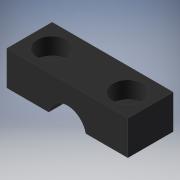
# Autodesk Inventor part: SHZA10-25_p
Saved by Autodesk Inventor 2019 (Build 230136000, 136)
## iProperties
Created: 2022-11-15
Part Number: SHZA10-25_p
Material: Generic
Catalog Web Link: www.cadenas.de
Description: SHZB, SHZM, SHZS, SHZA_p-Shaft Supports - Side Mount - Split Type
Vendor: MISUMI
Document SubType Name: Modeling
Designer: psAdmin
Manufacturer: MISUMI
Mass: 2.50843 g
Surface Area: 18.379 cm^2
Volume: 2.50843 cm^3
Density: 1 g/cm^3
Appearance: PSOLRGB-175-175-175
Category: PARTsolutions
Company: MISUMI
Title: SHZA10-25
Author: Cadenas PARTsolutions
Comments: Shaft Supports - Side Mount - Split Type
PSOL_IDENT_0: {$CADENAS_DATA/23d-libs/misumi/metric/02_shaft_supports/shzb_p.prj},200 {VTYP=3D},{NB=SHZA10-25_p},{
PSOL_IDENT_1: LINA=SHZA10-25},{NN=SHZB, SHZM, SHZS, SHZA_p},{DATE=30.07.2021 12:27:22},{GEOMDATE=30.08.2016 08:17:
PSOL_IDENT_2: 00},{VERSION=},{LINEID=60},{WBVAR=MAT,ST,HS,ALT1,HC},{WBNUMERIC=HS,HC}  {NB=SHZA10-25_p},{LINA=SHZA1
PSOL_IDENT_3: 0-25},{KT=DUMMY},{PN=SHZA10-25},{TYPE=SHZA},{MAT=6063},{ST=Clear Anodizing},{AC=Hexagon Socket Head
PSOL_IDENT_4: Cap Screw 1pc (Stainless Steel)},{D=10},{HS=25},{ALT1=-},{HC=0.0},{H=25.0},{L=32},{H1=35.0},{H2=5},{
PSOL_IDENT_5: TS=12},{T=12},{TA=12},{L1=20},{DD=4.5},{M=M4 Depth 8},{THMD=4},{THDMIN=3.242},{HCT=},{DEP=8},{DD1=8}
PSOL_IDENT_6: ,{DD2=4.5},{LL=4.5},{C=2.0},{HM=10.000},{H0=10},{HH=25,'25',30,'30'},{HC1=[25:30/0.1]},{HCA=0},{HPN=
PSOL_IDENT_7: -25},{ALTPN=},{HSALG=25,'25',30,'30'},{HCC1=0},{STA='Clear Anodizing','Clear Anodizing'}
NB: SHZA10-25_p
NN: SHZB, SHZM, SHZS, SHZA_p
NT: Shaft Supports - Side Mount - Split Type
NBSYN: $PN._p
LINA: SHZA10-25
CATALOG: Misumi
PN: SHZA10-25
MAT: 6063 Aluminum Alloy
ST: Clear Anodizing
D: 10
HS: 25
ALT1: w/o HC ( Mounting Height )
HC: 0
L: 32
H2: 5
TS: 12
TA: 12
L1: 20
DD: 4.5
M: M4 Depth 8
THMD: 4
THDMIN: 3.242
DEP: 8
DD1: 8
DD2: 4.5
LL: 4.5
C: 2
HM: 10
H0: 10
HH: 25,'25',30,'30'
HC1: [25:30/0.1]
SUPPLIER: MISUMI
ARTICLENO: SHZA10-25_p
BOMINFO: SHZA10-25
CREATOR: CADENAS GmbH
Autodesk Inventor part; units mm, degrees
sketch "Sketch_10" plane through (0, 0, 0) normal (0, 0, 1) x (1, 0, 0)
  line L0 (-16, 35) -> (-16, 26)
  line L1 (-16, 26) -> (-4.899, 26)
  arc A0 (4.899, 26) -> (-4.899, 26) centre (0, 25) ccw
  line L2 (4.899, 26) -> (16, 26)
  line L3 (16, 26) -> (16, 35)
  line L4 (16, 35) -> (-16, 35)
  constraints: 10 end point, 2 point on circle, 1 centre point
extrude "Extrusion1" add sketch "Sketch_10" along normal mid plane 12
sketch "Sketch2" plane through (-16, 35, 6) normal (0, 1, 0) x (1, 0, 0)
  point P0 (26, 6)
hole "Hole1" at (10, 35, 0) direction (0, -1, 0) diameter 4.5 depth 9 counterbore diameter 8 counterbore depth 4.5
sketch "Sketch3" plane through (-16, 35, 6) normal (0, 1, 0) x (1, 0, 0)
  point P0 (6, 6)
hole "Hole2" at (-10, 35, 0) direction (0, -1, 0) diameter 4.5 depth 9 counterbore diameter 8 counterbore depth 4.5
ref_plane "p_to_b_XY" through (0, 0, 0) normal (0, 1, 0) x (1, 0, 0)
ref_plane "p_to_b_YZ" through (0, 0, 0) normal (1, 0, 0) x (0, 0, -1)
ref_plane "p_to_b_ZX" through (0, 0, 0) normal (0, 0, -1) x (0, 1, 0)
body "Solid1"
